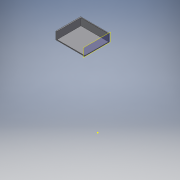
# Autodesk Inventor part: BatCap
Saved by Autodesk Inventor 2016 SP2 (Build 200236200, 236)
## iProperties
Created: 2018-06-21
Part Number: BatCap
Material: Generisch
Document SubType Name: Modeling
Designer: Nils
Density: 1 g/cm^3
Appearance: Vorgabe
Author: Nils
Autodesk Inventor part; units mm, degrees
ref_plane "YZ Plane" through (0, 0, 0) normal (1, 0, 0) x (0, 1, 0)
ref_plane "XZ Plane" through (0, 0, 0) normal (0, 1, 0) x (-1, 0, 0)
ref_plane "XY Plane" through (0, 0, 0) normal (0, 0, 1) x (1, 0, 0)
ref_plane "Arbeitsebene1" through (575.6121, -61.149, 338.1375) normal (-1, 0, 0) x (0, -1, 0)
sketch "Skizze1" plane through (575.6121, -61.149, 338.1375) normal (-1, 0, 0) x (0, -1, 0)
  line L0 (74, -2) -> (75, -1)
  line L1 (74, 0) -> (74, -2)
  line L2 (75, -3) -> (-7.5, -3)
  line L3 (-7.5, -3) -> (-7.5, 23)
  line L4 (-4.5, 22) -> (-3.5, 23)
  line L5 (-6.5, 22) -> (-4.5, 22)
  line L6 (-5.5, 23) -> (-6.5, 22)
  line L7 (-5.5, 23) -> (-7.5, 23)
  line L8 (75, -3) -> (75, -1)
  line L9 (74, -1) -> (-5.5, -1)
  line L10 (-5.5, -1) -> (-5.5, 22)
  point P0 (-61.149, -338.1375)
extrude "Extrusion1" add sketch "Skizze1" along normal blind 92.5
sketch "Skizze3" plane through (483.1121, -61.149, 338.1375) normal (-1, 0, 0) x (0, 0, 1)
  line L0 (-3, 7.5) -> (23, 7.5) projected
  line L1 (-3, -75) -> (23, -75)
  line L2 (23, -75) -> (23, 7.5)
  line L3 (23, 7.5) -> (-3, 7.5)
  line L4 (-3, 7.5) -> (-3, -75)
  point P0 (-338.1375, 61.149)
  constraints: 8 end point, 2 parallel, 1 coincident, 1 horizontal, 1 perpendicular, 1 other
extrude "Extrusion2" add sketch "Skizze3" along normal blind 3
